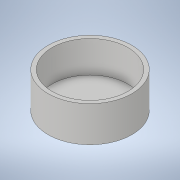
# Autodesk Inventor part: LargeFinderObjectiveCover
Saved by Autodesk Inventor 2021.1 (Build 251245000, 245)
## iProperties
Created: 2018-09-01
Part Number: LargeFinderObjectiveCover
Material: Generic
Document SubType Name: Modeling
Designer: steele
Density: 1 g/cm^3
Appearance: Default
Author: steele
Autodesk Inventor part; units mm, degrees
ref_plane "YZ Plane" through (0, 0, 0) normal (1, 0, 0) x (0, 1, 0)
ref_plane "XZ Plane" through (0, 0, 0) normal (0, 1, 0) x (-1, 0, 0)
ref_plane "XY Plane" through (0, 0, 0) normal (0, 0, 1) x (1, 0, 0)
sketch "Sketch1" plane through (0, 0, 0) normal (0, 1, 0) x (-1, 0, 0)
  circle A0 centre (0, 0) radius 33.655
  dimension "d0" = 67.31
  constraints: 1 centre point, 1 coincident
  measures "d0" diameter of A0
extrude "Extrusion1" add sketch "Sketch1" along normal blind 3.175
sketch "Sketch2" plane through (0, 3.175, 0) normal (0, 1, 0) x (1, 0, 0)
  circle A0 centre (0, 0) radius 33.655
  circle A1 centre (0, 0) radius 30.48
  dimension "d4" = 60.96
  dimension "d5" = 67.31
  constraints: 2 centre point, 1 coincident
  measures "d4" diameter of A1
  measures "d5" diameter of A0
extrude "Extrusion3" add sketch "Sketch2" along normal blind 25.4
equation "\"d0\" = lensCoverOD"
equation "\"d2\" = wallThickness"
equation "\"d4\" = lensCoverID"
equation "\"d5\" = lensCoverOD"
equation "\"d9\" = lensCoverLength"
equation "\"objectiveOD\" = 60.325"
equation "\"lensCoverLength\" = 25.4"
equation "\"wallThickness\" = 3.175"
equation "\"lensCoverOD\" = lensCoverID + 2 * wallThickness"
equation "\"clearance\" = 0.635"
equation "\"lensCoverID\" = objectiveOD + clearance"
body "Solid1"
